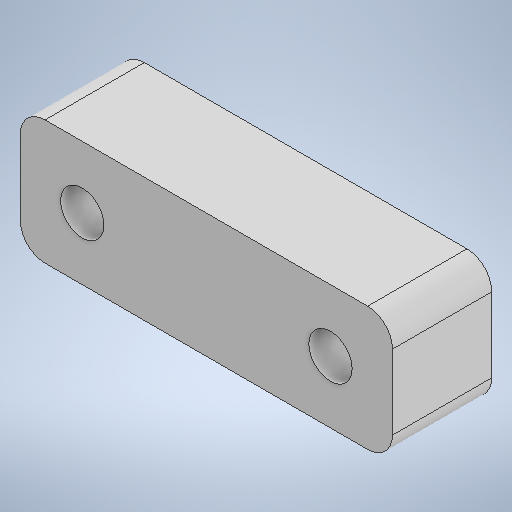
# Autodesk Inventor part: gear_enco_plate
Saved by Autodesk Inventor 2025.1 (Build 291241000, 241)
## iProperties
Created: 2024-12-11
Part Number: gear_enco_plate
Material: 一般
Document SubType Name: Modeling
Designer: yuki0520
Density: 1 g/cm^3
Appearance: 既定
Author: yuki0520
Autodesk Inventor part; units mm, degrees
ref_plane "YZ Plane" through (0, 0, 0) normal (1, 0, 0) x (0, 1, 0)
ref_plane "XZ Plane" through (0, 0, 0) normal (0, 1, 0) x (-1, 0, 0)
ref_plane "XY Plane" through (0, 0, 0) normal (0, 0, 1) x (1, 0, 0)
sketch "スケッチ1" plane through (0, 0, 0) normal (0, 0, 1) x (1, 0, 0)
  line L0 (15, -5) -> (-15, -5)
  line L1 (-15, -5) -> (-15, 5)
  line L2 (-15, 5) -> (15, 5)
  line L3 (15, 5) -> (15, -5)
  line L4 (15, -5) -> (-15, 5) construction
  line L5 (-15, -5) -> (15, 5) construction
  line L6 (-15, 0) -> (15, 0)
  circle A0 centre (-10, 0) radius 1.75
  circle A1 centre (10, 0) radius 1.75
  point P0 (0, 0)
  point P1 (0, 0)
  dimension "d0" = 30
  dimension "d1" = 10
  dimension "d2" = 3.5
  dimension "d3" = 3.5
  dimension "d4" = 20
  dimension "d5" = 10
  constraints: 14 end point, 5 midpoint, 2 centre point, 2 parallel, 2 point on line, 1 horizontal, 1 perpendicular
  measures "d0" distance of L1.end L2.end
  measures "d1" distance of L0.end L1.end
  measures "d2" diameter of A0
  measures "d3" diameter of A1
  measures "d4" distance of A1.centre A0.centre
  measures "d5" distance of point (0, 0) A1.centre
extrude "押し出し1" add sketch "スケッチ1" along normal blind 8 contours L0 L1 L6 A0 A1 L3 | L6 A1 A0 L1 L2 L3
fillet "フィレット1" radius 2 4 edges at (-15, 5, 4) (15, 5, 4) (15, -5, 4) (-15, -5, 4)
equation "\"d5\" = 0.5 * d4"
